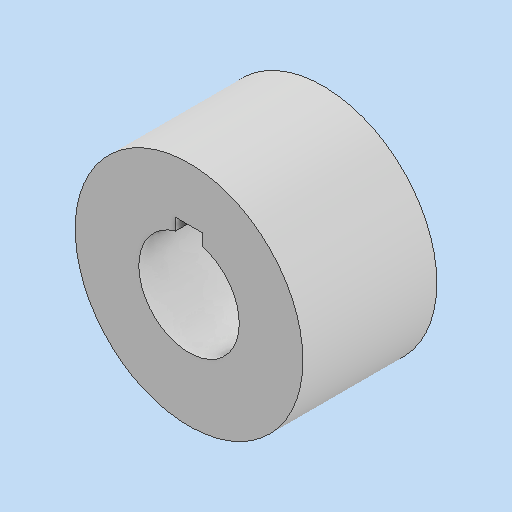
# Autodesk Inventor part: gear1
Saved by Autodesk Inventor 2022 (Build 260153000, 153)
## iProperties
Created: 2023-12-21
Part Number: gear1
Material: 一般
Document SubType Name: Modeling
Designer: ktamu
Density: 1 g/cm^3
Appearance: 既定
Author: ktamu
Autodesk Inventor part; units mm, degrees
ref_plane "YZ Plane" through (0, 0, 0) normal (1, 0, 0) x (0, 1, 0)
ref_plane "XZ Plane" through (0, 0, 0) normal (0, 1, 0) x (-1, 0, 0)
ref_plane "XY Plane" through (0, 0, 0) normal (0, 0, 1) x (1, 0, 0)
sketch "スケッチ1" plane through (0, 0, 0) normal (0, 0, 1) x (1, 0, 0)
  circle A0 centre (0, 0) radius 34
  arc A1 (-4, 14.4568) -> (4, 14.4568) centre (0, 0) ccw
  line L0 (0, 15) -> (0, 11)
  line L1 (0, 15) -> (0, 18)
  line L2 (0, 18) -> (4, 18)
  line L3 (4, 18) -> (4, 14.4568)
  line L4 (4, 11) -> (0, 11)
  line L5 (0, 18) -> (-4, 18)
  line L6 (-4, 18) -> (-4, 14.4568)
  line L7 (-4, 11) -> (0, 11)
  point P0 (-4, 14.5)
  point P1 (4, 14.5)
  dimension "d0" = 68
  dimension "d1" = 30
  dimension "d2" = 4
  dimension "d3" = 3
  dimension "d4" = 4
  constraints: 16 end point, 3 coincident, 2 centre point, 2 perpendicular, 2 point on circle, 2 point on line, 2 symmetric about line, 2 vertical, 1 horizontal
  measures "d0" diameter of A0
  measures "d1" diameter of A1
  measures "d2" distance of L0.start L0.end
  measures "d3" distance of L0.start L1.end
  measures "d4" distance of L1.end L2.end
extrude "押し出し1" add sketch "スケッチ1" along normal blind 40
